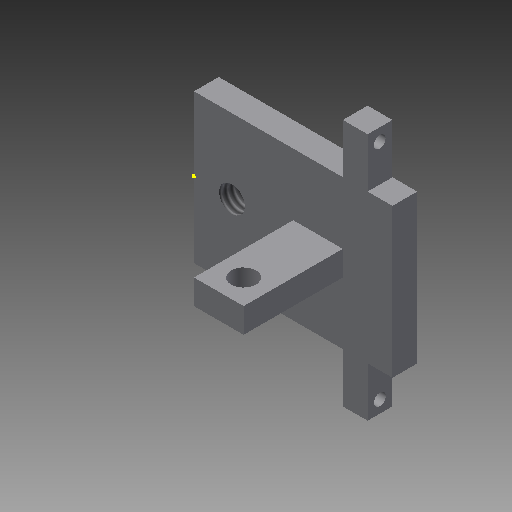
# Autodesk Inventor part: slide pivot plate
Saved by Autodesk Inventor 2017 (Build 210142000, 142)
## iProperties
Created: 2017-01-31
Part Number: slide pivot plate
Material: Generic
Document SubType Name: Modeling
Designer: Mark Koeppen
Density: 1 g/cm^3
Appearance: Default
Mass: 1.85645 g
Surface Area: 17.0797 cm^2
Volume: 1.85645 cm^3
Author: Mark Koeppen
Autodesk Inventor part; units mm, degrees
ref_plane "YZ Plane" through (0, 0, 0) normal (1, 0, 0) x (0, 1, 0)
ref_plane "XZ Plane" through (0, 0, 0) normal (0, 1, 0) x (-1, 0, 0)
ref_plane "XY Plane" through (0, 0, 0) normal (0, 0, 1) x (1, 0, 0)
sketch "Sketch1" plane through (0, 0, 0) normal (0, 0, 1) x (1, 0, 0)
  line L0 (0, -9.713) -> (25.4, -9.713)
  line L1 (25.4, -9.713) -> (25.4, 9.337)
  line L2 (0, 9.337) -> (0, -9.713)
  line L3 (19.05, 9.337) -> (19.05, 15.687)
  line L4 (19.05, 15.687) -> (22.225, 15.687)
  line L5 (22.225, 15.687) -> (22.225, 9.337)
  line L6 (25.4, 9.337) -> (22.225, 9.337)
  line L7 (19.05, 9.337) -> (0, 9.337)
  dimension "d0" = 19.05
  dimension "d2" = 25.4
  dimension "d3" = 3.175
  dimension "d4" = 6.35
  dimension "d22" = 3.175
  constraints: 16 end point, 4 parallel, 4 perpendicular, 1 collinear, 1 horizontal
  measures "d0" distance of L2.start L0.start
  measures "d2" distance of L1.end L2.start
  measures "d3" distance between parallel lines of L5 L3
  measures "d4" distance between parallel lines of L6 L4
  measures "d22" distance between parallel lines of L5 L1
extrude "Extrusion1" add sketch "Sketch1" against normal blind 3.175
sketch "Sketch2" plane through (0, 0, 0) normal (0, 0, 1) x (1, 0, 0)
  line L0 (12.7, -1.7755) -> (19.05, -1.7755)
  line L1 (19.05, -1.7755) -> (19.05, 1.3995)
  line L2 (19.05, 1.3995) -> (12.7, 1.3995)
  line L3 (12.7, 1.3995) -> (12.7, -1.7755)
  line L4 (0, 9.337) -> (0, -9.713) projected
  line L5 (25.4, 9.337) -> (22.225, 9.337) projected
  line L6 (25.4, -9.713) -> (25.4, 9.337) projected
  dimension "d7" = 3.175
  dimension "d10" = 6.35
  dimension "d11" = 7.9375
  dimension "d12" = 6.35
  constraints: 8 end point, 2 parallel, 1 horizontal, 1 perpendicular
  measures "d7" distance between parallel lines of L0 L2
  measures "d10" distance between parallel lines of L1 L3
  measures "d11" distance between parallel lines of L2 L5
  measures "d12" distance between parallel lines of L1 L6
extrude "Extrusion2" add sketch "Sketch2" along normal blind 12.7
sketch "Sketch3" plane through (22.225, 9.337, 0) normal (1, 0, 0) x (0, 0, -1)
  line L0 (0, 0) -> (0, 6.35) projected
  line L1 (0, 0) -> (3.175, 0) projected
  line L2 (3.175, 6.35) -> (3.175, 0) projected
  line L3 (0, 6.35) -> (3.175, 6.35) projected
  point P0 (1.5537, 4.7498)
  dimension "d38" = 1.6002
  measures "d38" distance from line of point (1.554, 4.75) L3
hole "Hole1" at (22.225, 14.0868, -1.5537) direction (-1, 0, 0) diameter 1.524 end through all
sketch "Sketch5" plane through (0, 0, -3.175) normal (0, 0, -1) x (-1, 0, 0)
  line L0 (-25.4, -9.713) -> (0, -9.713) projected
  line L1 (0, -9.713) -> (0, 9.337) projected
  line L2 (0, 9.337) -> (-19.05, 9.337) projected
  line L3 (-19.05, 9.337) -> (-19.05, 15.687) projected
  line L4 (-19.05, 15.687) -> (-22.225, 15.687) projected
  line L5 (-22.225, 15.687) -> (-22.225, 9.337) projected
  line L6 (-22.225, 9.337) -> (-25.4, 9.337) projected
  line L7 (-25.4, 9.337) -> (-25.4, -9.713) projected
  point P0 (-22.225, -11.491)
  point P1 (-4.8639, -0.1739)
  dimension "d37" = 3.175
  measures "d37" distance from line of point (-22.225, -11.491) L7
hole "Hole3" at (4.8639, -0.1739, -3.175) at (22.225, -11.491, -3.175) direction (0, 0, 1) diameter 3.302 end through all thread size "8-32 UNC" class "2B" standard "ANSI Unified Screw Threads"
sketch "Sketch6" plane through (22.225, 9.337, 0) normal (1, 0, 0) x (0, 0, -1)
  point P0 (0, -9.337)
sketch "Sketch7" plane through (0, 0, 0) normal (0, 0, 1) x (1, 0, 0)
  point P0 (0, 0)
sketch "Sketch8" plane through (0, -9.713, 0) normal (0, -1, 0) x (1, 0, 0)
  line L0 (25.4, 0) -> (22.225, 0) projected
  line L1 (22.225, 0) -> (22.225, -3.175) projected
  line L2 (19.05, -3.175) -> (22.225, -3.175) projected
  line L3 (0, 0) -> (25.4, 0) projected
  line L4 (22.225, -3.175) -> (25.4, -3.175) projected
  line L5 (22.225, -3.175) -> (19.05, -3.175)
  line L6 (19.05, -3.175) -> (19.05, 0)
  line L7 (19.05, 0) -> (22.225, 0)
  line L8 (22.225, 0) -> (22.225, -3.175)
  constraints: 8 end point, 2 parallel, 1 horizontal, 1 perpendicular, 1 point on line
extrude "Extrusion3" add sketch "Sketch8" along normal blind 6.35
hole "Hole4" at (19.05, -14.4755, -1.5875) direction (1, 0, 0) diameter 1.524 depth 25.4 tip angle 118
hole "Hole5" at (15.875, -1.7755, 9.525) direction (0, 1, 0) diameter 3.175 depth 25.4 tip angle 118
equation "\"d11\" = -0.5 * d7 + 0.5 * d0"
body "Solid1"
